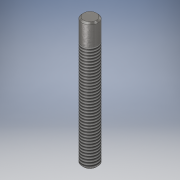
# Autodesk Inventor part: HVU_ignition_coil_studs
Saved by Autodesk Inventor 2017 (Build 210142000, 142)
## iProperties
Part Number: HVU_ignition_coil_studs
Material: Stahl, galvanisiert
Document SubType Name: Modeling
Designer: David Merges
Density: 7.85 g/cm^3
Appearance: Galvanisiert
Author: David Merges
Autodesk Inventor part; units mm, degrees
ref_plane "YZ Plane" through (0, 0, 0) normal (1, 0, 0) x (0, 1, 0)
ref_plane "XZ Plane" through (0, 0, 0) normal (0, 1, 0) x (-1, 0, 0)
ref_plane "XY Plane" through (0, 0, 0) normal (0, 0, 1) x (1, 0, 0)
sketch "Skizze1" plane through (0, 0, 0) normal (0, 0, 1) x (1, 0, 0)
  circle A0 centre (0, 0) radius 1.5
  dimension "d0" = 3
  constraints: 1 centre point, 1 coincident
  measures "d0" diameter of A0
extrude "Extrusion1" add sketch "Skizze1" along normal mid plane 24
thread "Gewinde2" size "M3x0.5" class "6g" standard "ANSI Metric M Profile" length 20
chamfer "Fase2" distance 0.3 angle 45 2 edges at (-1.5, 0, -12) (-1.5, 0, 12)
